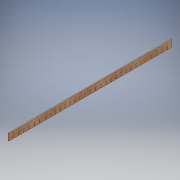
# Autodesk Inventor part: DividerLength
Saved by Autodesk Inventor 2016 (Build 200138000, 138)
## iProperties
Created: 2016-02-08
Part Number: DividerLength
Material: Wood (Birch)
Document SubType Name: Modeling
Designer: ron
Density: 0.55 g/cm^3
Appearance: Birch - Natural Polished
Author: ron
Autodesk Inventor part; units mm, degrees
ref_plane "YZ Plane" through (0, 0, 0) normal (1, 0, 0) x (0, 1, 0)
ref_plane "XZ Plane" through (0, 0, 0) normal (0, 1, 0) x (-1, 0, 0)
ref_plane "XY Plane" through (0, 0, 0) normal (0, 0, 1) x (1, 0, 0)
sketch "Sketch1" plane through (0, 0, 0) normal (1, 0, 0) x (0, 1, 0)
  line L0 (0, 0) -> (50.8, 0)
  line L1 (50.8, 0) -> (50.8, -1219.2)
  line L2 (50.8, -1219.2) -> (0, -1219.2)
  line L3 (0, -1219.2) -> (0, -1184.275)
  line L4 (0, -1184.275) -> (25.4, -1184.275)
  line L5 (25.4, -1184.275) -> (25.4, -1181.1)
  line L6 (22.225, -1177.925) -> (0, -1177.925)
  line L7 (0, -1177.925) -> (0, -1146.175)
  line L8 (0, -1146.175) -> (25.4, -1146.175)
  line L9 (25.4, -1146.175) -> (25.4, -1139.825)
  line L10 (25.4, -1139.825) -> (0, -1139.825)
  line L11 (0, -1139.825) -> (0, -1108.075)
  line L12 (0, -1108.075) -> (25.4, -1108.075)
  line L13 (25.4, -1108.075) -> (25.4, -1101.725)
  line L14 (25.4, -1101.725) -> (0, -1101.725)
  line L15 (0, -1101.725) -> (0, -1069.975)
  line L16 (0, -1069.975) -> (25.4, -1069.975)
  line L17 (25.4, -1069.975) -> (25.4, -1063.625)
  line L18 (25.4, -1063.625) -> (0, -1063.625)
  line L19 (0, -1063.625) -> (0, -1031.875)
  line L20 (0, -1031.875) -> (25.4, -1031.875)
  line L21 (25.4, -1031.875) -> (25.4, -1025.525)
  line L22 (25.4, -1025.525) -> (0, -1025.525)
  line L23 (0, -1025.525) -> (0, -993.775)
  line L24 (0, -993.775) -> (25.4, -993.775)
  line L25 (25.4, -993.775) -> (25.4, -987.425)
  line L26 (25.4, -987.425) -> (0, -987.425)
  line L27 (0, -987.425) -> (0, -955.675)
  line L28 (0, -955.675) -> (25.4, -955.675)
  line L29 (25.4, -955.675) -> (25.4, -949.325)
  line L30 (25.4, -949.325) -> (0, -949.325)
  line L31 (0, -949.325) -> (0, -917.575)
  line L32 (0, -917.575) -> (25.4, -917.575)
  line L33 (25.4, -917.575) -> (25.4, -911.225)
  line L34 (25.4, -911.225) -> (0, -911.225)
  line L35 (0, -911.225) -> (0, -879.475)
  line L36 (0, -879.475) -> (25.4, -879.475)
  line L37 (25.4, -879.475) -> (25.4, -873.125)
  line L38 (25.4, -873.125) -> (0, -873.125)
  line L39 (0, -873.125) -> (0, -841.375)
  line L40 (0, -841.375) -> (25.4, -841.375)
  line L41 (25.4, -841.375) -> (25.4, -835.025)
  line L42 (25.4, -835.025) -> (0, -835.025)
  line L43 (0, -835.025) -> (0, -803.275)
  line L44 (0, -803.275) -> (25.4, -803.275)
  line L45 (25.4, -803.275) -> (25.4, -796.925)
  line L46 (25.4, -796.925) -> (0, -796.925)
  line L47 (0, -796.925) -> (0, -765.175)
  line L48 (0, -765.175) -> (25.4, -765.175)
  line L49 (25.4, -765.175) -> (25.4, -758.825)
  line L50 (25.4, -758.825) -> (0, -758.825)
  line L51 (0, -758.825) -> (0, -727.075)
  line L52 (0, -727.075) -> (25.4, -727.075)
  line L53 (25.4, -727.075) -> (25.4, -720.725)
  line L54 (25.4, -720.725) -> (0, -720.725)
  line L55 (0, -720.725) -> (0, -688.975)
  line L56 (0, -688.975) -> (25.4, -688.975)
  line L57 (25.4, -688.975) -> (25.4, -682.625)
  line L58 (25.4, -682.625) -> (0, -682.625)
  line L59 (0, -682.625) -> (0, -650.875)
  line L60 (0, -650.875) -> (25.4, -650.875)
  line L61 (25.4, -650.875) -> (25.4, -644.525)
  line L62 (25.4, -644.525) -> (0, -644.525)
  line L63 (0, -644.525) -> (0, -612.775)
  line L64 (0, -612.775) -> (25.4, -612.775)
  line L65 (25.4, -612.775) -> (25.4, -606.425)
  line L66 (25.4, -606.425) -> (0, -606.425)
  line L67 (0, -606.425) -> (0, -574.675)
  line L68 (0, -574.675) -> (25.4, -574.675)
  line L69 (25.4, -574.675) -> (25.4, -568.325)
  line L70 (25.4, -568.325) -> (0, -568.325)
  line L71 (0, -568.325) -> (0, -536.575)
  line L72 (0, -536.575) -> (25.4, -536.575)
  line L73 (25.4, -536.575) -> (25.4, -530.225)
  line L74 (25.4, -530.225) -> (0, -530.225)
  line L75 (0, -530.225) -> (0, -498.475)
  line L76 (0, -498.475) -> (25.4, -498.475)
  line L77 (25.4, -498.475) -> (25.4, -492.125)
  line L78 (25.4, -492.125) -> (0, -492.125)
  line L79 (0, -492.125) -> (0, -460.375)
  line L80 (0, -460.375) -> (25.4, -460.375)
  line L81 (25.4, -460.375) -> (25.4, -454.025)
  line L82 (25.4, -454.025) -> (0, -454.025)
  line L83 (0, -454.025) -> (0, -422.275)
  line L84 (0, -422.275) -> (25.4, -422.275)
  line L85 (25.4, -422.275) -> (25.4, -415.925)
  line L86 (25.4, -415.925) -> (0, -415.925)
  line L87 (0, -415.925) -> (0, -384.175)
  line L88 (0, -384.175) -> (25.4, -384.175)
  line L89 (25.4, -384.175) -> (25.4, -377.825)
  line L90 (25.4, -377.825) -> (0, -377.825)
  line L91 (0, -377.825) -> (0, -346.075)
  line L92 (0, -346.075) -> (25.4, -346.075)
  line L93 (25.4, -346.075) -> (25.4, -339.725)
  line L94 (25.4, -339.725) -> (0, -339.725)
  line L95 (0, -339.725) -> (0, -307.975)
  line L96 (0, -307.975) -> (25.4, -307.975)
  line L97 (25.4, -307.975) -> (25.4, -301.625)
  line L98 (25.4, -301.625) -> (0, -301.625)
  line L99 (0, -301.625) -> (0, -269.875)
  line L100 (0, -269.875) -> (25.4, -269.875)
  line L101 (25.4, -269.875) -> (25.4, -263.525)
  line L102 (25.4, -263.525) -> (0, -263.525)
  line L103 (0, -263.525) -> (0, -231.775)
  line L104 (0, -231.775) -> (25.4, -231.775)
  line L105 (25.4, -231.775) -> (25.4, -225.425)
  line L106 (25.4, -225.425) -> (0, -225.425)
  line L107 (0, -225.425) -> (0, -193.675)
  line L108 (0, -193.675) -> (25.4, -193.675)
  line L109 (25.4, -193.675) -> (25.4, -187.325)
  line L110 (25.4, -187.325) -> (0, -187.325)
  line L111 (0, -187.325) -> (0, -155.575)
  line L112 (0, -155.575) -> (25.4, -155.575)
  line L113 (25.4, -155.575) -> (25.4, -149.225)
  line L114 (25.4, -149.225) -> (0, -149.225)
  line L115 (0, -149.225) -> (0, -117.475)
  line L116 (0, -117.475) -> (25.4, -117.475)
  line L117 (25.4, -117.475) -> (25.4, -111.125)
  line L118 (25.4, -111.125) -> (0, -111.125)
  line L119 (0, -111.125) -> (0, -79.375)
  line L120 (0, -79.375) -> (25.4, -79.375)
  line L121 (25.4, -79.375) -> (25.4, -73.025)
  line L122 (25.4, -73.025) -> (0, -73.025)
  line L123 (0, -73.025) -> (0, -41.275)
  line L124 (0, -41.275) -> (25.4, -41.275)
  line L125 (25.4, -41.275) -> (25.4, -34.925)
  line L126 (25.4, -34.925) -> (0, -34.925)
  line L127 (0, -34.925) -> (0, 0)
  line L128 (22.225, -1177.925) -> (25.4, -1177.925)
  line L129 (25.4, -1177.925) -> (25.4, -1181.1)
  dimension "d209" = 25.4
  dimension "d210" = 25.4
  dimension "d211" = 25.4
  dimension "d212" = 25.4
  dimension "d213" = 25.4
  dimension "d214" = 25.4
  dimension "d215" = 25.4
  dimension "d216" = 25.4
  dimension "d217" = 25.4
  dimension "d218" = 25.4
  dimension "d219" = 25.4
  dimension "d220" = 25.4
  dimension "d221" = 25.4
  dimension "d222" = 25.4
  dimension "d223" = 25.4
  dimension "d224" = 25.4
  dimension "d225" = 50.8
  dimension "d226" = 1219.2
  dimension "d227" = 1177.925
  dimension "d228" = 34.925
  dimension "d229" = 41.275
  dimension "d230" = 73.025
  dimension "d231" = 79.375
  dimension "d232" = 111.125
  dimension "d233" = 117.475
  dimension "d234" = 149.225
  dimension "d235" = 155.575
  dimension "d236" = 187.325
  dimension "d237" = 193.675
  dimension "d238" = 225.425
  dimension "d239" = 231.775
  dimension "d240" = 263.525
  dimension "d241" = 269.875
  dimension "d242" = 301.625
  dimension "d243" = 307.975
  dimension "d244" = 339.725
  dimension "d245" = 346.075
  dimension "d246" = 377.825
  dimension "d247" = 384.175
  dimension "d248" = 415.925
  dimension "d249" = 422.275
  dimension "d250" = 454.025
  dimension "d251" = 460.375
  dimension "d252" = 492.125
  dimension "d253" = 498.475
  dimension "d254" = 530.225
  dimension "d255" = 536.575
  dimension "d256" = 568.325
  dimension "d257" = 574.675
  dimension "d258" = 606.425
  dimension "d259" = 612.775
  dimension "d260" = 644.525
  dimension "d261" = 650.875
  dimension "d262" = 682.625
  dimension "d263" = 688.975
  dimension "d264" = 720.725
  dimension "d265" = 727.075
  dimension "d266" = 758.825
  dimension "d267" = 765.175
  dimension "d268" = 796.925
  dimension "d269" = 803.275
  dimension "d270" = 835.025
  dimension "d271" = 841.375
  dimension "d272" = 873.125
  constraints: 261 end point, 79 point on line, 65 perpendicular, 31 parallel, 1 collinear, 1 horizontal
  measures "d209" distance between parallel lines of L1 L125
  measures "d210" distance between parallel lines of L1 L117
  measures "d211" distance between parallel lines of L113 L1
  measures "d212" distance between parallel lines of L105 L1
  measures "d213" distance between parallel lines of L97 L1
  measures "d214" distance between parallel lines of L89 L1
  measures "d215" distance between parallel lines of L81 L1
  measures "d216" distance between parallel lines of L73 L1
  measures "d217" distance between parallel lines of L65 L1
  measures "d218" distance between parallel lines of L57 L1
  measures "d219" distance between parallel lines of L49 L1
  measures "d220" distance between parallel lines of L41 L1
  measures "d221" distance between parallel lines of L33 L1
  measures "d222" distance between parallel lines of L25 L1
  measures "d223" distance between parallel lines of L17 L1
  measures "d224" distance between parallel lines of L1 L5
  measures "d225" distance between parallel lines of L1 L3
  measures "d226" distance between parallel lines of L0 L2
  measures "d227" distance between parallel lines of L128 L0
  measures "d228" distance between parallel lines of L0 L126
  measures "d229" distance between parallel lines of L0 L124
  measures "d230" distance between parallel lines of L0 L122
  measures "d231" distance between parallel lines of L0 L120
  measures "d232" distance between parallel lines of L0 L118
  measures "d233" distance between parallel lines of L0 L116
  measures "d234" distance between parallel lines of L0 L114
  measures "d235" distance between parallel lines of L0 L112
  measures "d236" distance between parallel lines of L0 L110
  measures "d237" distance between parallel lines of L0 L108
  measures "d238" distance between parallel lines of L0 L106
  measures "d239" distance between parallel lines of L0 L104
  measures "d240" distance between parallel lines of L0 L102
  measures "d241" distance between parallel lines of L0 L100
  measures "d242" distance between parallel lines of L0 L98
  measures "d243" distance between parallel lines of L0 L96
  measures "d244" distance between parallel lines of L0 L94
  measures "d245" distance between parallel lines of L0 L92
  measures "d246" distance between parallel lines of L0 L90
  measures "d247" distance between parallel lines of L0 L88
  measures "d248" distance between parallel lines of L0 L86
  measures "d249" distance between parallel lines of L0 L84
  measures "d250" distance between parallel lines of L0 L82
  measures "d251" distance between parallel lines of L0 L80
  measures "d252" distance between parallel lines of L0 L78
  measures "d253" distance between parallel lines of L0 L76
  measures "d254" distance between parallel lines of L0 L74
  measures "d255" distance between parallel lines of L0 L72
  measures "d256" distance between parallel lines of L0 L70
  measures "d257" distance between parallel lines of L0 L68
  measures "d258" distance between parallel lines of L0 L66
  measures "d259" distance between parallel lines of L0 L64
  measures "d260" distance between parallel lines of L0 L62
  measures "d261" distance between parallel lines of L0 L60
  measures "d262" distance between parallel lines of L0 L58
  measures "d263" distance between parallel lines of L0 L56
  measures "d264" distance between parallel lines of L0 L54
  measures "d265" distance between parallel lines of L0 L52
  measures "d266" distance between parallel lines of L0 L50
  measures "d267" distance between parallel lines of L0 L48
  measures "d268" distance between parallel lines of L0 L46
  measures "d269" distance between parallel lines of L0 L44
  measures "d270" distance between parallel lines of L0 L42
  measures "d271" distance between parallel lines of L0 L40
  measures "d272" distance between parallel lines of L0 L38
extrude "Extrusion1" add sketch "Sketch1" along normal blind 6.35
body "Solid1"
